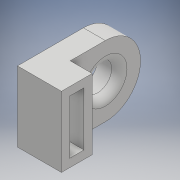
# Autodesk Inventor part: frameAdjustment 11-28
Saved by Autodesk Inventor 2018 (Build 220112000, 112)
## iProperties
Created: 2019-11-28
Part Number: frameAdjustment 11-28
Material: Generic
Document SubType Name: Modeling
Designer: Aditya Kendre
Density: 1 g/cm^3
Appearance: Default
Author: Aditya Kendre
Autodesk Inventor part; units mm, degrees
ref_plane "YZ Plane" through (0, 0, 0) normal (1, 0, 0) x (0, 1, 0)
ref_plane "XZ Plane" through (0, 0, 0) normal (0, 1, 0) x (-1, 0, 0)
ref_plane "XY Plane" through (0, 0, 0) normal (0, 0, 1) x (1, 0, 0)
sketch "Sketch1" plane through (0, 0, 0) normal (1, 0, 0) x (0, 1, 0)
  line L0 (0, 0) -> (3.25, 0)
  line L1 (3.25, 0) -> (3.25, -12.25)
  line L2 (3.25, -12.25) -> (0, -12.25)
  line L3 (0, -12.25) -> (0, 0)
  line L4 (-1.875, -14.125) -> (5.125, -14.125)
  line L5 (5.125, -14.125) -> (5.125, 1.875)
  line L6 (5.125, 1.875) -> (-1.875, 1.875)
  line L7 (-1.875, 1.875) -> (-1.875, -14.125)
  line L8 (-1.875, -14.125) -> (5.125, 1.875) construction
  line L9 (5.125, -14.125) -> (-1.875, 1.875) construction
  point P0 (1.625, -6.125)
  dimension "d0" = 3.25
  dimension "d1" = 12.25
  dimension "d2" = 7
  dimension "d3" = 16
  constraints: 20 end point, 4 parallel, 2 horizontal, 2 midpoint, 2 perpendicular
  measures "d0" distance of L1.end L2.end
  measures "d1" distance of L0.end L1.end
  measures "d2" distance of L6.end L5.end
  measures "d3" distance of L5.end L4.end
extrude "Extrusion1" add sketch "Sketch1" along normal blind 10
sketch "Sketch2" plane through (0, 5.125, 1.875) normal (0, 1, 0) x (1, 0, 0)
  line L0 (0, 0) -> (0, 16) projected
  line L1 (0, 16) -> (10, 16) projected
  line L2 (0, 0) -> (5, 0)
  line L3 (5, 0) -> (5, 16)
  line L4 (5, 16) -> (0, 16)
  line L5 (0, 16) -> (0, 0)
  point P0 (0, 1.875)
  dimension "d6" = 5
  constraints: 8 end point, 2 parallel, 1 horizontal, 1 midpoint, 1 perpendicular
  measures "d6" distance of L4.end L3.end
extrude "Extrusion2" add sketch "Sketch2" along normal blind 16
sketch "Sketch3" plane through (5, 5.125, 1.875) normal (1, 0, 0) x (0, 0, -1)
  line L0 (16, 0) -> (0, 0) construction
  line L1 (0, -7) -> (0, 16) construction
  line L2 (16, 0) -> (0, 16) construction
  circle A0 centre (8, 8) radius 3.175
  point P0 (1.875, -5.125)
  dimension "d9" = 6.35
  constraints: 2 end point, 1 centre point, 1 midpoint
  measures "d9" diameter of A0
extrude "Extrusion3" cut sketch "Sketch3" against normal blind 16
fillet "Fillet1" radius 8 2 edges at (2.5, 21.125, 1.875) (2.5, 21.125, -14.125)
fillet "Fillet2" radius 1.75 1 edges at (5, 13.125, -2.95)
body "Solid1"
